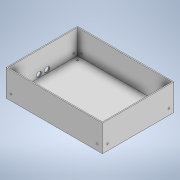
# Autodesk Inventor part: Lower Chassis_2
Saved by Autodesk Inventor 2020 (Build 240168000, 168)
## iProperties
Created: 2021-12-09
Part Number: Lower Chassis_2
Material: Generic
Document SubType Name: Modeling
Designer: danie
Density: 1 g/cm^3
Appearance: Default
Author: danie
Autodesk Inventor part; units mm, degrees
ref_plane "YZ Plane" through (0, 0, 0) normal (1, 0, 0) x (0, 1, 0)
ref_plane "XZ Plane" through (0, 0, 0) normal (0, 1, 0) x (-1, 0, 0)
ref_plane "XY Plane" through (0, 0, 0) normal (0, 0, 1) x (1, 0, 0)
sketch "Sketch1" plane through (0, 0, 0) normal (0, 1, 0) x (-1, 0, 0)
  line L0 (0, 0) -> (-299.72, 0)
  line L1 (-299.72, 0) -> (-299.72, 222.25)
  line L2 (-299.72, 222.25) -> (0, 222.25)
  line L3 (0, 222.25) -> (0, 0)
  dimension "d0" = 299.72
  dimension "d1" = 222.25
  constraints: 8 end point, 2 parallel, 1 horizontal, 1 perpendicular
  measures "d0" distance of L1.end L2.end
  measures "d1" distance of L0.end L1.end
extrude "Extrusion1" add sketch "Sketch1" along normal blind 6.35
sketch "Sketch2" plane through (0, 6.35, 0) normal (0, 1, 0) x (1, 0, 0)
  line L0 (0, 0) -> (0, -222.25) projected
  line L1 (299.72, -222.25) -> (299.72, 0) projected
  line L2 (0, -222.25) -> (299.72, -222.25)
  line L3 (299.72, -222.25) -> (299.72, 0)
  line L4 (299.72, 0) -> (0, 0)
  line L5 (0, 0) -> (0, -222.25)
  line L6 (296.545, -219.075) -> (3.175, -219.075)
  line L7 (3.175, -219.075) -> (3.175, -3.175)
  line L8 (3.175, -3.175) -> (296.545, -3.175)
  line L9 (296.545, -3.175) -> (296.545, -219.075)
  point P0 (299.72, -222.25)
  dimension "d4" = 3.175
  constraints: 16 end point, 4 parallel, 2 perpendicular, 1 horizontal, 3 other
  measures "d4" distance between parallel lines of L2 L6
extrude "Extrusion2" add sketch "Sketch2" along normal blind 76.2
sketch "Sketch3" plane through (0, 6.35, 0) normal (0, 1, 0) x (1, 0, 0)
  line L0 (3.175, -219.075) -> (3.175, -3.175) construction
  line L1 (3.175, -3.175) -> (28.575, -3.175) construction
  line L2 (28.575, -3.175) -> (28.575, -28.575) construction
  line L3 (28.575, -28.575) -> (3.175, -28.575) construction
  line L4 (3.175, -28.575) -> (3.175, -3.175) construction
  line L5 (296.545, -3.175) -> (271.145, -3.175) construction
  line L6 (271.145, -3.175) -> (271.145, -28.575) construction
  line L7 (271.145, -28.575) -> (296.545, -28.575) construction
  line L8 (296.545, -28.575) -> (296.545, -3.175) construction
  line L9 (296.545, -219.075) -> (3.175, -219.075) construction
  line L10 (296.545, -219.075) -> (271.145, -219.075) construction
  line L11 (271.145, -219.075) -> (271.145, -193.675) construction
  line L12 (271.145, -193.675) -> (296.545, -193.675) construction
  line L13 (296.545, -193.675) -> (296.545, -219.075) construction
  line L14 (3.175, -219.075) -> (28.575, -219.075) construction
  line L15 (28.575, -219.075) -> (28.575, -193.675) construction
  line L16 (28.575, -193.675) -> (3.175, -193.675) construction
  line L17 (3.175, -193.675) -> (3.175, -219.075) construction
  line L18 (3.175, -193.675) -> (28.575, -219.075) construction
  line L19 (28.575, -193.675) -> (3.175, -219.075) construction
  line L20 (271.145, -193.675) -> (296.545, -219.075) construction
  line L21 (296.545, -219.075) -> (296.545, -193.675) construction
  line L22 (296.545, -193.675) -> (271.145, -219.075) construction
  line L23 (271.145, -3.175) -> (296.545, -28.575) construction
  line L24 (296.545, -3.175) -> (271.145, -28.575) construction
  line L25 (3.175, -3.175) -> (28.575, -28.575) construction
  line L26 (28.575, -3.175) -> (3.175, -28.575) construction
  circle A0 centre (15.875, -15.875) radius 2.3812
  circle A1 centre (283.845, -15.875) radius 2.3812
  circle A2 centre (283.845, -206.375) radius 2.3812
  circle A3 centre (15.875, -206.375) radius 2.3813
  point P0 (0, 0)
  dimension "d7" = 25.4
  dimension "d8" = 25.4
  dimension "d9" = 25.4
  dimension "d10" = 25.4
  dimension "d11" = 25.4
  dimension "d12" = 25.4
  dimension "d13" = 25.4
  dimension "d14" = 25.4
  dimension "d15" = 4.7625
  dimension "d16" = 4.7625
  dimension "d17" = 4.7625
  dimension "d18" = 4.7625
  constraints: 50 end point, 9 equal length, 4 centre point, 4 horizontal, 4 midpoint, 4 perpendicular
  measures "d7" distance of L2.end L3.end
  measures "d8" distance of L1.end L2.end
  measures "d9" distance of L7.end L6.end
  measures "d10" distance of L6.end L5.end
  measures "d11" distance of L11.end L12.end
  measures "d12" distance of L10.end L11.end
  measures "d13" distance of L16.end L15.end
  measures "d14" distance of L15.end L14.end
  measures "d15" diameter of A0
  measures "d16" diameter of A1
  measures "d17" diameter of A2
  measures "d18" diameter of A3
extrude "Extrusion3" cut sketch "Sketch3" against normal blind 6.35
sketch "Sketch4" plane through (3.175, 6.35, 219.075) normal (1, 0, 0) x (0, 0, -1)
  line L0 (215.9, 0) -> (0, 0) construction
  line L1 (0, 0) -> (25.4, 0) construction
  line L2 (25.4, 0) -> (25.4, 25.4) construction
  line L3 (25.4, 25.4) -> (0, 25.4) construction
  line L4 (0, 25.4) -> (0, 0) construction
  line L5 (215.9, 0) -> (190.5, 0) construction
  line L6 (190.5, 0) -> (190.5, 25.4) construction
  line L7 (190.5, 25.4) -> (215.9, 25.4) construction
  line L8 (215.9, 25.4) -> (215.9, 0) construction
  line L9 (0, 25.4) -> (25.4, 0) construction
  line L10 (25.4, 25.4) -> (0, 0) construction
  line L11 (190.5, 25.4) -> (215.9, 0) construction
  line L12 (215.9, 25.4) -> (190.5, 0) construction
  circle A0 centre (203.2, 12.7) radius 2.3813
  circle A1 centre (12.7, 12.7) radius 2.3813
  point P0 (219.075, -6.35)
  dimension "d21" = 25.4
  dimension "d22" = 25.4
  dimension "d23" = 25.4
  dimension "d24" = 25.4
  dimension "d25" = 4.7625
  dimension "d26" = 4.7625
  constraints: 24 end point, 4 parallel, 2 centre point, 2 horizontal, 2 midpoint, 2 perpendicular
  measures "d21" distance of L3.end L2.end
  measures "d22" distance of L2.end L1.end
  measures "d23" distance of L6.end L7.end
  measures "d24" distance of L5.end L6.end
  measures "d25" diameter of A0
  measures "d26" diameter of A1
extrude "Extrusion4" cut sketch "Sketch4" against normal blind 3.175
sketch "Sketch5" plane through (3.175, 6.35, 3.175) normal (0, 0, 1) x (1, 0, 0)
  line L0 (0, 0) -> (0, 76.2) construction
  line L1 (0, 0) -> (25.4, 0) construction
  line L2 (25.4, 0) -> (25.4, 25.4) construction
  line L3 (25.4, 25.4) -> (0, 25.4) construction
  line L4 (0, 25.4) -> (0, 0) construction
  line L5 (293.37, 0) -> (267.97, 0) construction
  line L6 (267.97, 0) -> (267.97, 25.4) construction
  line L7 (267.97, 25.4) -> (293.37, 25.4) construction
  line L8 (293.37, 25.4) -> (293.37, 0) construction
  line L9 (0, 25.4) -> (25.4, 0) construction
  line L10 (293.37, 0) -> (0, 0) construction
  line L11 (25.4, 25.4) -> (0, 0) construction
  line L12 (293.37, 25.4) -> (267.97, 0) construction
  line L13 (293.37, 0) -> (293.37, 76.2) construction
  line L14 (267.97, 25.4) -> (293.37, 0) construction
  circle A0 centre (280.67, 12.7) radius 2.3812
  circle A1 centre (12.7, 12.7) radius 2.3813
  point P0 (-3.175, -6.35)
  dimension "d29" = 25.4
  dimension "d30" = 25.4
  dimension "d31" = 25.4
  dimension "d32" = 25.4
  dimension "d33" = 4.7625
  dimension "d34" = 4.7625
  constraints: 24 end point, 4 parallel, 2 centre point, 2 horizontal, 2 midpoint, 2 perpendicular
  measures "d29" distance of L3.end L2.end
  measures "d30" distance of L2.end L1.end
  measures "d31" distance of L6.end L7.end
  measures "d32" distance of L5.end L6.end
  measures "d33" diameter of A0
  measures "d34" diameter of A1
extrude "Extrusion5" cut sketch "Sketch5" against normal blind 3.175
sketch "Sketch6" plane through (296.545, 6.35, 3.175) normal (-1, 0, 0) x (0, 0, 1)
  line L0 (215.9, 0) -> (0, 0) construction
  line L1 (0, 0) -> (25.4, 0) construction
  line L2 (25.4, 0) -> (25.4, 25.4) construction
  line L3 (25.4, 25.4) -> (0, 25.4) construction
  line L4 (0, 25.4) -> (0, 0) construction
  line L5 (215.9, 0) -> (190.5, 0) construction
  line L6 (190.5, 0) -> (190.5, 25.4) construction
  line L7 (190.5, 25.4) -> (215.9, 25.4) construction
  line L8 (215.9, 25.4) -> (215.9, 0) construction
  line L9 (190.5, 0) -> (215.9, 25.4) construction
  line L10 (215.9, 0) -> (215.9, 76.2) construction
  line L11 (190.5, 25.4) -> (215.9, 0) construction
  line L12 (0, 25.4) -> (25.4, 0) construction
  line L13 (25.4, 25.4) -> (0, 0) construction
  circle A0 centre (12.7, 12.7) radius 2.3812
  circle A1 centre (203.2, 12.7) radius 2.3813
  point P0 (-3.175, -6.35)
  dimension "d37" = 25.4
  dimension "d38" = 25.4
  dimension "d39" = 25.4
  dimension "d40" = 25.4
  dimension "d41" = 4.7625
  dimension "d42" = 4.7625
  constraints: 24 end point, 4 parallel, 2 centre point, 2 horizontal, 2 midpoint, 2 perpendicular
  measures "d37" distance of L3.end L2.end
  measures "d38" distance of L2.end L1.end
  measures "d39" distance of L6.end L7.end
  measures "d40" distance of L5.end L6.end
  measures "d41" diameter of A0
  measures "d42" diameter of A1
extrude "Extrusion6" cut sketch "Sketch6" against normal blind 3.175
sketch "Sketch7" plane through (296.545, 6.35, 219.075) normal (0, 0, -1) x (-1, 0, 0)
  line L0 (293.37, 0) -> (267.97, 0) construction
  line L1 (267.97, 0) -> (267.97, 25.4) construction
  line L2 (267.97, 25.4) -> (293.37, 25.4) construction
  line L3 (293.37, 25.4) -> (293.37, 0) construction
  line L4 (293.37, 0) -> (0, 0) construction
  line L5 (0, 0) -> (25.4, 0) construction
  line L6 (25.4, 0) -> (25.4, 25.4) construction
  line L7 (25.4, 25.4) -> (0, 25.4) construction
  line L8 (0, 25.4) -> (0, 0) construction
  line L9 (0, 25.4) -> (25.4, 0) construction
  line L10 (25.4, 25.4) -> (0, 0) construction
  line L11 (267.97, 0) -> (293.37, 25.4) construction
  line L12 (267.97, 25.4) -> (293.37, 0) construction
  circle A0 centre (280.67, 12.7) radius 2.3812
  circle A1 centre (12.7, 12.7) radius 2.3813
  point P0 (296.545, -6.35)
  dimension "d45" = 25.4
  dimension "d46" = 25.4
  dimension "d47" = 25.4
  dimension "d48" = 25.4
  dimension "d49" = 4.7625
  dimension "d50" = 4.7625
  constraints: 24 end point, 4 parallel, 2 centre point, 2 horizontal, 2 midpoint, 2 perpendicular
  measures "d45" distance of L1.end L2.end
  measures "d46" distance of L0.end L1.end
  measures "d47" distance of L7.end L6.end
  measures "d48" distance of L6.end L5.end
  measures "d49" diameter of A0
  measures "d50" diameter of A1
extrude "Extrusion7" cut sketch "Sketch7" against normal blind 3.175
sketch "Sketch8" plane through (3.175, 6.35, 219.075) normal (1, 0, 0) x (0, 0, -1)
  line L0 (215.9, 0) -> (0, 0) construction
  line L1 (0, 0) -> (107.95, 0) construction
  line L2 (107.95, 0) -> (130.175, 0) construction
  line L3 (107.95, 0) -> (130.175, 0) construction
  line L4 (130.175, 0) -> (85.725, 0) construction
  line L5 (85.725, 0) -> (85.725, 20.6375) construction
  line L6 (85.725, 20.6375) -> (130.175, 20.6375) construction
  line L7 (130.175, 20.6375) -> (130.175, 0) construction
  line L8 (85.725, 0) -> (85.725, 10.3251) construction
  line L9 (130.175, 0) -> (130.175, 10.3251) construction
  line L10 (130.175, 0) -> (140.5001, 0) construction
  line L11 (85.725, 10.3251) -> (87.3125, 10.3251) construction
  line L12 (130.175, 10.3251) -> (128.5875, 10.3251) construction
  line L13 (128.5875, 10.3251) -> (120.65, 10.3251) construction
  line L14 (128.5875, 10.3251) -> (136.525, 10.3251) construction
  line L15 (87.3125, 10.3251) -> (95.25, 10.3251) construction
  line L16 (87.3125, 10.3251) -> (95.25, 10.3251) construction
  circle A0 centre (95.25, 10.3251) radius 7.9375
  circle A1 centre (120.65, 10.3251) radius 7.9375
  dimension "d53" = 107.95
  dimension "d54" = 22.225
  dimension "d55" = 0
  dimension "d56" = 44.45
  dimension "d57" = 20.6375
  dimension "d58" = 10.3251
  dimension "d59" = 10.3251
  dimension "d60" = 90
  dimension "d61" = 1.5875
  dimension "d62" = 1.5875
  dimension "d64" = 7.9375
  dimension "d65" = 180
  dimension "d66" = 7.9375
  dimension "d67" = 0
  dimension "d68" = 15.875
  dimension "d69" = 15.875
  constraints: 32 end point, 9 horizontal, 4 equal length, 2 centre point, 2 coincident, 2 parallel, 1 collinear, 1 midpoint, 1 perpendicular, 1 point on line, 1 vertical
  measures "d53" distance of L0.end L1.end
  measures "d54" distance of L1.end L2.end
  measures "d55" distance between parallel lines of L2 L3
  measures "d56" distance of L5.end L6.end
  measures "d57" distance of L4.end L5.end
  measures "d58" distance of L4.end L8.end
  measures "d59" distance of L3.end L9.end
  measures "d60" angle of L10 L9
  measures "d61" distance of L8.end L11.end
  measures "d62" distance of L9.end L12.end
  measures "d64" distance of L12.end L13.end
  measures "d65" angle of L13 L14
  measures "d66" distance of L11.end L15.end
  measures "d67" distance between parallel lines of L15 L16
  measures "d68" diameter of A0
  measures "d69" diameter of A1
extrude "Extrusion8" cut sketch "Sketch8" against normal blind 3.175
body "Solid1"
